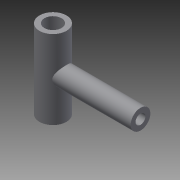
# Autodesk Inventor part: WagonAttachementV04
Saved by Autodesk Inventor 2014 (Build 180170000, 170)
## iProperties
Created: 2013-11-25
Part Number: WagonAttachementV04
Material: Generic
Document SubType Name: Modeling
Designer: steele
Density: 1 g/cm^3
Appearance: Default
Author: steele
Autodesk Inventor part; units mm, degrees
ref_plane "XZ Plane" through (0, 0, 0) normal (0, 1, 0) x (-1, 0, 0)
sketch "Sketch1" plane through (0, 0, 0) normal (0, 0, 1) x (1, 0, 0)
  circle A0 centre (0, 0) radius 17.3736
  circle A1 centre (0, 0) radius 11.0236
  dimension "d0" = 34.7472
  dimension "d1" = 22.0472
  constraints: 2 centre point, 2 coincident
  measures "d0" diameter of A0
  measures "d1" diameter of A1
extrude "Extrusion1" add sketch "Sketch1" along normal mid plane 101.6
ref_plane "Work Plane1" through (11.2776, 0, 0) normal (1, 0, 0) x (0, 1, 0)
sketch "Sketch2" plane through (11.2776, 0, 0) normal (1, 0, 0) x (0, 1, 0)
  circle A0 centre (0, 0) radius 12.7
  circle A1 centre (0, 0) radius 6.35
  dimension "d5" = 25.4
  dimension "d8" = 12.7
  constraints: 2 centre point, 2 coincident
  measures "d5" diameter of A0
  measures "d8" diameter of A1
extrude "Extrusion3" add sketch "Sketch2" along normal blind 101.6
ref_plane "Work Plane2" through (-21.5, 0, 0) normal (1, 0, 0) x (0, 1, 0)
sketch "Sketch7" plane through (-21.5, 0, 0) normal (1, 0, 0) x (0, 1, 0)
  line L0 (4, 56) -> (4, -56) construction
  line L1 (-4, 36.2853) -> (4, 38.295)
  line L2 (4, 38.295) -> (4, 39.4878)
  line L3 (4, 39.4878) -> (-2.6386, 41.1151)
  line L4 (-2.6386, 41.1151) -> (4, 42.6969)
  line L5 (4, 42.6969) -> (4, 43.8768)
  line L6 (4, 43.8768) -> (-4, 45.919)
  line L7 (-4, 45.919) -> (-4, 44.8233)
  line L8 (-4, 44.8233) -> (2.6321, 43.2156)
  line L9 (2.6321, 43.2156) -> (-4, 41.6207)
  line L10 (-4, 41.6207) -> (-4, 40.5381)
  line L11 (-4, 40.5381) -> (2.7099, 38.9303)
  line L12 (2.7099, 38.9303) -> (-4, 37.329)
  line L13 (-4, 37.329) -> (-4, 36.2853)
  spline S0 degree 2 poles (3.3647, 32.0648) (3.4554, 32.188) (3.7796, 32.6029) (3.8768, 32.7974) knots 0 0 0 1 2 2 2
  spline S1 degree 2 poles (3.8768, 32.7974) (4.0194, 33.0632) (4.1686, 33.5624) (4.1686, 34.0162) knots 0 0 0 1 2 2 2
  spline S2 degree 2 poles (4.1686, 34.0162) (4.1686, 34.3857) (3.8898, 35.0535) (3.637, 35.3063) knots 0 0 0 1 2 2 2
  spline S3 degree 2 poles (3.637, 35.3063) (3.3906, 35.5462) (2.6645, 35.8379) (2.2626, 35.8379) knots 0 0 0 1 2 2 2
  spline S4 degree 2 poles (2.2626, 35.8379) (1.6402, 35.8379) (0.7585, 35.3128) (0.5057, 34.7423) knots 0 0 0 1 2 2 2
  spline S5 degree 2 poles (0.5057, 34.7423) (0.2723, 34.2366) (0.0972, 32.8622) (0.0519, 32.0648) knots 0 0 0 1 2 2 2
  line L14 (0.0519, 32.0648) -> (-0.1426, 32.0648)
  spline S6 degree 2 poles (-0.1426, 32.0648) (-0.4927, 32.0648) (-0.9271, 32.2788) (-1.0502, 32.4733) knots 0 0 0 1 2 2 2
  spline S7 degree 2 poles (-1.0502, 32.4733) (-1.1734, 32.6678) (-1.2512, 33.2253) (-1.2512, 33.5235) knots 0 0 0 1 2 2 2
  spline S8 degree 2 poles (-1.2512, 33.5235) (-1.2512, 33.8736) (-1.0438, 34.8201) (-0.8428, 35.2934) knots 0 0 0 1 2 2 2
  line L15 (-0.8428, 35.2934) -> (-0.8428, 35.3517)
  line L16 (-0.8428, 35.3517) -> (-1.8736, 35.3517)
  spline S9 degree 2 poles (-1.8736, 35.3517) (-1.9514, 35.0729) (-2.1459, 34.0292) (-2.1459, 33.517) knots 0 0 0 1 2 2 2
  spline S10 degree 2 poles (-2.1459, 33.517) (-2.1459, 32.8947) (-1.9514, 32.0454) (-1.6985, 31.7083) knots 0 0 0 1 2 2 2
  spline S11 degree 2 poles (-1.6985, 31.7083) (-1.4522, 31.3776) (-0.6677, 31.0535) (-0.1037, 31.0535) knots 0 0 0 1 2 2 2
  line L17 (-0.1037, 31.0535) -> (4, 31.0535)
  line L18 (4, 31.0535) -> (4, 32.0648)
  line L19 (4, 32.0648) -> (3.3647, 32.0648)
  line L20 (2.5219, 32.0648) -> (0.8558, 32.0648)
  spline S12 degree 2 poles (0.8558, 32.0648) (0.8882, 32.4279) (0.9984, 33.5235) (1.1021, 33.8671) knots 0 0 0 1 2 2 2
  spline S13 degree 2 poles (1.1021, 33.8671) (1.2253, 34.269) (1.7374, 34.7942) (2.1912, 34.7942) knots 0 0 0 1 2 2 2
  spline S14 degree 2 poles (2.1912, 34.7942) (2.7099, 34.7942) (3.235, 34.2107) (3.235, 33.6532) knots 0 0 0 1 2 2 2
  spline S15 degree 2 poles (3.235, 33.6532) (3.235, 33.1799) (2.8266, 32.4019) (2.5219, 32.0648) knots 0 0 0 1 2 2 2
  spline S16 degree 2 poles (4.9595, 29.4198) (5.0049, 29.316) (5.1475, 28.9206) (5.2058, 28.6678) knots 0 0 0 1 2 2 2
  spline S17 degree 2 poles (5.2058, 28.6678) (5.2771, 28.389) (5.3614, 27.9157) (5.3614, 27.637) knots 0 0 0 1 2 2 2
  spline S18 degree 2 poles (5.3614, 27.637) (5.3614, 27.1702) (5.1151, 26.5219) (4.8947, 26.3404) knots 0 0 0 1 2 2 2
  spline S19 degree 2 poles (4.8947, 26.3404) (4.6742, 26.1653) (4.0972, 26.0292) (3.7277, 26.0292) knots 0 0 0 1 2 2 2
  line L21 (3.7277, 26.0292) -> (3.2026, 26.0292)
  spline S20 degree 2 poles (3.2026, 26.0292) (3.5592, 26.4376) (3.8963, 27.222) (3.8963, 27.812) knots 0 0 0 1 2 2 2
  spline S21 degree 2 poles (3.8963, 27.812) (3.8963, 28.8363) (2.3728, 30.0486) (0.94, 30.0486) knots 0 0 0 1 2 2 2
  spline S22 degree 2 poles (0.94, 30.0486) (0.1945, 30.0486) (-0.9595, 29.6272) (-1.3679, 29.2772) knots 0 0 0 1 2 2 2
  spline S23 degree 2 poles (-1.3679, 29.2772) (-1.7504, 28.94) (-2.1718, 28.013) (-2.1718, 27.5203) knots 0 0 0 1 2 2 2
  spline S24 degree 2 poles (-2.1718, 27.5203) (-2.1718, 27.0535) (-1.9514, 26.3728) (-1.7504, 26.0292) knots 0 0 0 1 2 2 2
  line L22 (-1.7504, 26.0292) -> (-2.0032, 25.9708)
  line L23 (-2.0032, 25.9708) -> (-2.0032, 25.0178)
  line L24 (-2.0032, 25.0178) -> (3.3128, 25.0178)
  spline S25 degree 2 poles (3.3128, 25.0178) (4.8428, 25.0178) (6.269, 26.3468) (6.269, 27.7148) knots 0 0 0 1 2 2 2
  spline S26 degree 2 poles (6.269, 27.7148) (6.269, 28.1556) (6.1264, 29.0762) (6.0097, 29.4716) knots 0 0 0 1 2 2 2
  line L25 (6.0097, 29.4716) -> (4.9595, 29.4716)
  line L26 (4.9595, 29.4716) -> (4.9595, 29.4198)
  line L27 (2.3728, 26.0292) -> (-0.9271, 26.0292)
  spline S27 degree 2 poles (-0.9271, 26.0292) (-1.1086, 26.4052) (-1.2642, 27.0405) (-1.2642, 27.3582) knots 0 0 0 1 2 2 2
  spline S28 degree 2 poles (-1.2642, 27.3582) (-1.2642, 28.1232) (-0.1361, 29.0049) (0.9206, 29.0049) knots 0 0 0 1 2 2 2
  spline S29 degree 2 poles (0.9206, 29.0049) (1.919, 29.0049) (2.9627, 28.3371) (2.9627, 27.5851) knots 0 0 0 1 2 2 2
  spline S30 degree 2 poles (2.9627, 27.5851) (2.9627, 27.1896) (2.6515, 26.3598) (2.3728, 26.0292) knots 0 0 0 1 2 2 2
  spline S31 degree 2 poles (0.9984, 18.6191) (2.5154, 18.6191) (4.1686, 20.0778) (4.1686, 21.2966) knots 0 0 0 1 2 2 2
  spline S32 degree 2 poles (4.1686, 21.2966) (4.1686, 22.5478) (2.4635, 23.9806) (0.9984, 23.9806) knots 0 0 0 1 2 2 2
  spline S33 degree 2 poles (0.9984, 23.9806) (-0.5057, 23.9806) (-2.1718, 22.5024) (-2.1718, 21.2966) knots 0 0 0 1 2 2 2
  spline S34 degree 2 poles (-2.1718, 21.2966) (-2.1718, 20.0778) (-0.5122, 18.6191) (0.9984, 18.6191) knots 0 0 0 1 2 2 2
  spline S35 degree 2 poles (0.9984, 19.6629) (-0.1686, 19.6629) (-1.3031, 20.5122) (-1.3031, 21.2966) knots 0 0 0 1 2 2 2
  spline S36 degree 2 poles (-1.3031, 21.2966) (-1.3031, 22.081) (-0.1686, 22.9368) (0.9984, 22.9368) knots 0 0 0 1 2 2 2
  spline S37 degree 2 poles (0.9984, 22.9368) (2.1329, 22.9368) (3.2998, 22.081) (3.2998, 21.2966) knots 0 0 0 1 2 2 2
  spline S38 degree 2 poles (3.2998, 21.2966) (3.2998, 20.5186) (2.1524, 19.6629) (0.9984, 19.6629) knots 0 0 0 1 2 2 2
  line L28 (4, 12.8687) -> (4, 13.8801)
  line L29 (4, 13.8801) -> (0.577, 13.8801)
  spline S39 degree 2 poles (0.577, 13.8801) (0.1621, 13.8801) (-0.5511, 13.9579) (-0.765, 14.0746) knots 0 0 0 1 2 2 2
  spline S40 degree 2 poles (-0.765, 14.0746) (-0.9919, 14.1977) (-1.2123, 14.6386) (-1.2123, 15.0146) knots 0 0 0 1 2 2 2
  spline S41 degree 2 poles (-1.2123, 15.0146) (-1.2123, 15.3906) (-0.8104, 16.188) (-0.4862, 16.5705) knots 0 0 0 1 2 2 2
  line L30 (-0.4862, 16.5705) -> (4, 16.5705)
  line L31 (4, 16.5705) -> (4, 17.5819)
  line L32 (4, 17.5819) -> (-2.0032, 17.5819)
  line L33 (-2.0032, 17.5819) -> (-2.0032, 16.5705)
  line L34 (-2.0032, 16.5705) -> (-1.3355, 16.5705)
  spline S42 degree 2 poles (-1.3355, 16.5705) (-1.7439, 16.1167) (-2.1718, 15.2415) (-2.1718, 14.7488) knots 0 0 0 1 2 2 2
  spline S43 degree 2 poles (-2.1718, 14.7488) (-2.1718, 13.8671) (-1.0049, 12.8687) (0.1037, 12.8687) knots 0 0 0 1 2 2 2
  line L35 (0.1037, 12.8687) -> (4, 12.8687)
  line L36 (4, 3.2998) -> (4, 7.9352)
  line L37 (4, 7.9352) -> (-4, 7.9352)
  line L38 (-4, 7.9352) -> (-4, 6.872)
  line L39 (-4, 6.872) -> (3.0535, 6.872)
  line L40 (3.0535, 6.872) -> (3.0535, 3.2998)
  line L41 (3.0535, 3.2998) -> (4, 3.2998)
  spline S44 degree 2 poles (0.9984, -2.3922) (2.5154, -2.3922) (4.1686, -0.9335) (4.1686, 0.2853) knots 0 0 0 1 2 2 2
  spline S45 degree 2 poles (4.1686, 0.2853) (4.1686, 1.5365) (2.4635, 2.9692) (0.9984, 2.9692) knots 0 0 0 1 2 2 2
  spline S46 degree 2 poles (0.9984, 2.9692) (-0.5057, 2.9692) (-2.1718, 1.4911) (-2.1718, 0.2853) knots 0 0 0 1 2 2 2
  spline S47 degree 2 poles (-2.1718, 0.2853) (-2.1718, -0.9335) (-0.5122, -2.3922) (0.9984, -2.3922) knots 0 0 0 1 2 2 2
  spline S48 degree 2 poles (0.9984, -1.3485) (-0.1686, -1.3485) (-1.3031, -0.4992) (-1.3031, 0.2853) knots 0 0 0 1 2 2 2
  spline S49 degree 2 poles (-1.3031, 0.2853) (-1.3031, 1.0697) (-0.1686, 1.9254) (0.9984, 1.9254) knots 0 0 0 1 2 2 2
  spline S50 degree 2 poles (0.9984, 1.9254) (2.1329, 1.9254) (3.2998, 1.0697) (3.2998, 0.2853) knots 0 0 0 1 2 2 2
  spline S51 degree 2 poles (3.2998, 0.2853) (3.2998, -0.4927) (2.1524, -1.3485) (0.9984, -1.3485) knots 0 0 0 1 2 2 2
  line L42 (-2.0032, -10.7034) -> (4, -9.1799)
  line L43 (4, -9.1799) -> (4, -8.2464)
  line L44 (4, -8.2464) -> (-0.6288, -6.7812)
  line L45 (-0.6288, -6.7812) -> (4, -5.3225)
  line L46 (4, -5.3225) -> (4, -4.3955)
  line L47 (4, -4.3955) -> (-2.0032, -2.859)
  line L48 (-2.0032, -2.859) -> (-2.0032, -3.9092)
  line L49 (-2.0032, -3.9092) -> (2.6451, -4.9724)
  line L50 (2.6451, -4.9724) -> (-2.0032, -6.3922)
  line L51 (-2.0032, -6.3922) -> (-2.0032, -7.2285)
  line L52 (-2.0032, -7.2285) -> (2.6451, -8.6872)
  line L53 (2.6451, -8.6872) -> (-2.0032, -9.6856)
  line L54 (-2.0032, -9.6856) -> (-2.0032, -10.7034)
  spline S52 degree 2 poles (4.1361, -14.1977) (4.1361, -12.7585) (2.5219, -11.1767) (1.0308, -11.1767) knots 0 0 0 1 2 2 2
  spline S53 degree 2 poles (1.0308, -11.1767) (-0.4344, -11.1767) (-2.1718, -12.7131) (-2.1718, -13.9514) knots 0 0 0 1 2 2 2
  spline S54 degree 2 poles (-2.1718, -13.9514) (-2.1718, -14.5089) (-1.8477, -15.3711) (-1.5041, -15.6888) knots 0 0 0 1 2 2 2
  spline S55 degree 2 poles (-1.5041, -15.6888) (-1.1605, -16.013) (-0.1686, -16.3566) (0.5511, -16.3566) knots 0 0 0 1 2 2 2
  line L55 (0.5511, -16.3566) -> (1.1021, -16.3566)
  line L56 (1.1021, -16.3566) -> (1.1021, -12.201)
  spline S56 degree 2 poles (1.1021, -12.201) (2.1459, -12.201) (3.2545, -13.2512) (3.2545, -14.1848) knots 0 0 0 1 2 2 2
  spline S57 degree 2 poles (3.2545, -14.1848) (3.2545, -14.5154) (3.1053, -15.1572) (2.9887, -15.4165) knots 0 0 0 1 2 2 2
  spline S58 degree 2 poles (2.9887, -15.4165) (2.859, -15.6888) (2.6321, -16.0648) (2.5284, -16.188) knots 0 0 0 1 2 2 2
  line L57 (2.5284, -16.188) -> (2.5284, -16.2464)
  line L58 (2.5284, -16.2464) -> (3.6305, -16.2464)
  spline S59 degree 2 poles (3.6305, -16.2464) (3.7018, -16.0713) (3.9092, -15.5397) (3.9676, -15.3323) knots 0 0 0 1 2 2 2
  spline S60 degree 2 poles (3.9676, -15.3323) (4.0519, -15.0405) (4.1361, -14.5608) (4.1361, -14.1977) knots 0 0 0 1 2 2 2
  spline S61 degree 2 poles (0.3306, -15.3711) (-0.0778, -15.3582) (-0.6742, -15.1896) (-0.8752, -15.0276) knots 0 0 0 1 2 2 2
  spline S62 degree 2 poles (-0.8752, -15.0276) (-1.1021, -14.8525) (-1.342, -14.3015) (-1.342, -13.893) knots 0 0 0 1 2 2 2
  spline S63 degree 2 poles (-1.342, -13.893) (-1.342, -13.4911) (-1.1021, -12.9271) (-0.8687, -12.6937) knots 0 0 0 1 2 2 2
  spline S64 degree 2 poles (-0.8687, -12.6937) (-0.6288, -12.4668) (-0.0519, -12.2334) (0.3306, -12.201) knots 0 0 0 1 2 2 2
  line L59 (0.3306, -12.201) -> (0.3306, -15.3711)
  line L60 (-0.9206, -20.564) -> (-0.9206, -20.5122)
  spline S65 degree 2 poles (-0.9206, -20.5122) (-0.953, -20.3955) (-0.966, -20.1426) (-0.966, -19.9676) knots 0 0 0 1 2 2 2
  spline S66 degree 2 poles (-0.966, -19.9676) (-0.966, -19.5592) (-0.6094, -18.7553) (-0.2593, -18.3922) knots 0 0 0 1 2 2 2
  line L61 (-0.2593, -18.3922) -> (4, -18.3922)
  line L62 (4, -18.3922) -> (4, -17.3809)
  line L63 (4, -17.3809) -> (-2.0032, -17.3809)
  line L64 (-2.0032, -17.3809) -> (-2.0032, -18.3922)
  line L65 (-2.0032, -18.3922) -> (-1.1086, -18.3922)
  spline S67 degree 2 poles (-1.1086, -18.3922) (-1.6013, -18.9433) (-2.0032, -19.7666) (-2.0032, -20.1556) knots 0 0 0 1 2 2 2
  spline S68 degree 2 poles (-2.0032, -20.1556) (-2.0032, -20.3112) (-1.9903, -20.4668) (-1.9708, -20.564) knots 0 0 0 1 2 2 2
  line L66 (-1.9708, -20.564) -> (-0.9206, -20.564)
  line L67 (-4, -30.6645) -> (4, -27.9092)
  line L68 (4, -27.9092) -> (4, -26.7617)
  line L69 (4, -26.7617) -> (-4, -24.0065)
  line L70 (-4, -24.0065) -> (-4, -25.1475)
  line L71 (-4, -25.1475) -> (2.6451, -27.3647)
  line L72 (2.6451, -27.3647) -> (-4, -29.5818)
  line L73 (-4, -29.5818) -> (-4, -30.6645)
  spline S69 degree 2 poles (0, -39.7083) (2.1524, -39.7083) (4.1686, -38.457) (4.1686, -37.154) knots 0 0 0 1 2 2 2
  spline S70 degree 2 poles (4.1686, -37.154) (4.1686, -35.8314) (2.1135, -34.5932) (0.0065, -34.5932) knots 0 0 0 1 2 2 2
  spline S71 degree 2 poles (0.0065, -34.5932) (-2.1588, -34.5932) (-4.1621, -35.8444) (-4.1621, -37.154) knots 0 0 0 1 2 2 2
  spline S72 degree 2 poles (-4.1621, -37.154) (-4.1621, -38.47) (-2.0875, -39.7083) (0, -39.7083) knots 0 0 0 1 2 2 2
  spline S73 degree 2 poles (2.4376, -38.3339) (2.0421, -38.4895) (0.8233, -38.6191) (0, -38.6191) knots 0 0 0 1 2 2 2
  spline S74 degree 2 poles (0, -38.6191) (-0.8233, -38.6191) (-2.0357, -38.4895) (-2.4441, -38.3274) knots 0 0 0 1 2 2 2
  spline S75 degree 2 poles (-2.4441, -38.3274) (-2.8525, -38.1653) (-3.2739, -37.6013) (-3.2739, -37.154) knots 0 0 0 1 2 2 2
  spline S76 degree 2 poles (-3.2739, -37.154) (-3.2739, -36.7066) (-2.8525, -36.1297) (-2.4311, -35.9611) knots 0 0 0 1 2 2 2
  spline S77 degree 2 poles (-2.4311, -35.9611) (-2.0227, -35.799) (-0.778, -35.6823) (0.0065, -35.6823) knots 0 0 0 1 2 2 2
  spline S78 degree 2 poles (0.0065, -35.6823) (0.8493, -35.6823) (1.9773, -35.7861) (2.4182, -35.9546) knots 0 0 0 1 2 2 2
  spline S79 degree 2 poles (2.4182, -35.9546) (2.8331, -36.1102) (3.2804, -36.6872) (3.2804, -37.154) knots 0 0 0 1 2 2 2
  spline S80 degree 2 poles (3.2804, -37.154) (3.2804, -37.5948) (2.859, -38.1718) (2.4376, -38.3339) knots 0 0 0 1 2 2 2
  line L74 (1.2512, -45.8801) -> (1.2512, -44.9271)
  line L75 (1.2512, -44.9271) -> (4, -44.9271)
  line L76 (4, -44.9271) -> (4, -43.8963)
  line L77 (4, -43.8963) -> (1.2512, -43.8963)
  line L78 (1.2512, -43.8963) -> (1.2512, -40.363)
  line L79 (1.2512, -40.363) -> (0.1232, -40.363)
  line L80 (0.1232, -40.363) -> (-4, -43.9417)
  line L81 (-4, -43.9417) -> (-4, -44.9271)
  line L82 (-4, -44.9271) -> (0.389, -44.9271)
  line L83 (0.389, -44.9271) -> (0.389, -45.8801)
  line L84 (0.389, -45.8801) -> (1.2512, -45.8801)
  line L85 (0.389, -43.8963) -> (-2.7358, -43.8963)
  line L86 (-2.7358, -43.8963) -> (0.389, -41.2058)
  line L87 (0.389, -41.2058) -> (0.389, -43.8963)
  point P0 (0, 0)
  dimension "d13" = 4
  constraints: 2 end point, 2 vertical
  measures "d13" distance from line of point (0, 0) L0
emboss "Emboss1" sketch "Sketch7" operation cut depth 1 direction (-1, 0, 0) wrap yes faces at (8.2071, -15.3129, 0)
body "Solid1"
